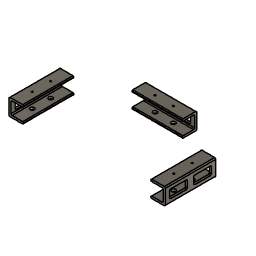
mac-holder v4 (Autodesk Fusion 360 design; units mm, degrees)
Autodesk Fusion 360 part; units mm, degrees
sketch "mac" plane through (0, 0, 0) normal (0, 0, 1) x (1, 0, 0)
  line L0 (0, 0) -> (355.6, 0)
  line L1 (355.6, 0) -> (355.6, 247.65)
  line L2 (355.6, 247.65) -> (0, 247.65)
  line L3 (0, 247.65) -> (0, 0)
  dimension "d1" = 355.6
  dimension "d2" = 247.65
  constraint horizontal L0
  constraint vertical L1
  constraint horizontal L2
  constraint vertical L3
  constraint coincident L0.start L3.end
  measures "d1" distance of L0.start L0.end
  measures "d2" distance of L0.start L2.end
extrude "Extrude1" add sketch "mac" along normal blind 19.05 makes body 1
sketch "front" plane through (0, 0, 0) normal (0, 1, 0) x (1, 0, 0)
  line L0 (0, 0) -> (0, -40)
  line L1 (0, -40) -> (35, -40)
  line L2 (35, -40) -> (35, -35)
  line L3 (35, -35) -> (5, -35)
  line L4 (5, -35) -> (5, -5)
  line L5 (5, -5) -> (35, -5)
  line L6 (35, -5) -> (35, 0)
  line L7 (35, 0) -> (0, 0)
  dimension "d5" = 5
  dimension "d6" = 5
  dimension "d7" = 5
  dimension "d8" = 30
  dimension "d9" = 35
  dimension "d10" = 35
  constraint coincident L0.start L7.end
  constraint vertical L0
  constraint perpendicular L0 L1
  constraint perpendicular L1 L2
  constraint perpendicular L0 L3
  constraint perpendicular L3 L4
  constraint perpendicular L4 L5
  constraint perpendicular L5 L6
  constraint perpendicular L0 L7
  measures "d5" distance of L5.end L6.end
  measures "d6" distance of L1.end L2.end
  measures "d7" distance of L0 L4
  measures "d8" distance of L3 L5
  measures "d9" distance of L6.end L0.start
  measures "d10" distance of L0.end L1.end
extrude "Extrude2" add sketch "front" along normal blind 120 separate body makes body 2
sketch "side" plane through (0, 0, 0) normal (-1, 0, 0) x (0, -1, 0)
  line L0 (0, 0) -> (0, 40)
  line L1 (0, 40) -> (-120, 40)
  line L2 (-120, 40) -> (-120, 0)
  line L3 (-120, 0) -> (0, 0)
  line L4 (-110, 10) -> (-10, 10)
  line L5 (-10, 10) -> (-10, 30)
  line L6 (-10, 30) -> (-110, 30)
  line L7 (-110, 30) -> (-110, 10)
  line L8 (-60, 30) -> (-60, 10) construction
  line L9 (-67.5, 30) -> (-67.5, 10)
  line L10 (-52.5, 30) -> (-52.5, 10)
  dimension "d13" = -10
  dimension "d14" = 7.5
  constraint midpoint L6 L8.start
  constraint midpoint L4 L8.end
  constraint coincident L6 L9.start
  constraint coincident L4 L9.end
  constraint perpendicular L4 L9
  constraint symmetric L8 L9.start L10.start
  constraint symmetric L8 L9.end L10.end
  measures "d14" distance of L8 L9
extrude "Extrude3" cut sketch "side" against normal up to surface (5 mm away) contours L4 L6 L7 L9 | L4 L5 L6 L10 bodies 2
fillet "Fillet1" radius 2.5 8 edges at (2.5, 52.5, 30) (2.5, 10, 30) (2.5, 10, 10) (2.5, 52.5, 10) (2.5, 67.5, 10) (2.5, 67.5, 30) (2.5, 110, 30) (2.5, 110, 10) on bodies 2
fillet "Fillet2" radius 2.5 2 edges at (0, 60, 40) (0, 60, 0) on bodies 2
fillet "Fillet3" radius 2.5 2 edges at (5, 60, 35) (5, 60, 5) on bodies 2
fillet "Fillet4" radius 2 4 edges at (35, 60, 40) (35, 60, 35) (35, 60, 5) (35, 60, 0) on bodies 2
sketch "top" plane through (0, 0, 40) normal (0, 0, 1) x (-1, 0, 0)
  line L0 (-33, 0) -> (-33, -120)
  line L1 (-33, -120) -> (-2.5, -120)
  line L2 (-2.5, -120) -> (-2.5, 0)
  line L3 (-2.5, 0) -> (-33, 0)
  line L4 (-33, -60) -> (-2.5, -60) construction
  line L5 (-17.75, -120) -> (-17.75, 0) construction
  circle A0 centre (-17.75, -38) radius 2
  circle A1 centre (-17.75, -82) radius 2
  circle A2 centre (-17.75, -38) radius 5
  circle A3 centre (-17.75, -82) radius 5
  circle A4 centre (-17.75, -38) radius 3
  circle A5 centre (-17.75, -82) radius 3
  dimension "d27" = 4
  dimension "d28" = 20
  dimension "d29" = 10
  dimension "d35" = 6
  constraint midpoint L0 L4.start
  constraint midpoint L2 L4.end
  constraint midpoint L1 L5.start
  constraint midpoint L3 L5.end
  constraint coincident L5 A0.centre
  constraint symmetric L4 A0 A1
  constraint concentric A0 A2
  constraint symmetric L4 A2 A3
  constraint concentric A0 A4
  constraint symmetric L4 A4 A5
  measures "d27" diameter of A0
  measures "d28" distance of L4 A0
  measures "d29" diameter of A2
  measures "d35" diameter of A4
extrude "Extrude4" cut sketch "top" against normal up to surface (40 mm away) contours A0 | A1 bodies 2
extrude "Extrude5" cut sketch "top" against normal up to surface (5 mm away) from surface at -35 contours A2 | A3 | A4 | A5 bodies 2
extrude "Extrude6" cut sketch "top" along normal blind 2 from surface at -5 contours A4 | A5 bodies 2
move_body "Move1" bodies 1 to x (1, 0, 0) y (0, 1, 0) z (0, 0, 1) at (9, 0, 10)
ref_plane "WorkPlane1" through (186.8, 123.825, 19.525) normal (1, 0, 0) x (0, 1, 0)
mirror "Mirror1" about plane through (186.8, 123.825, 19.525) normal (1, 0, 0) of bodies 2 makes body 3
fillet "Fillet5" radius 10 4 edges at (9, 0, 19.525) (364.6, 0, 19.525) (364.6, 247.65, 19.525) (9, 247.65, 19.525) on bodies 1
move_body "Move2" bodies 1 to x (1, 0, 0) y (0, 1, 0) z (0, 0, 1) at (0, -60, 0)
copy_body "CopyPasteBodies1" bodies 3 makes body 4
move_body "Move3" bodies 4 to x (0, 1, 0) y (-1, 0, 0) z (0, 0, 1) at (258.6, -178.6, 0)
move_body "Move4" bodies 4 to x (1, 0, 0) y (0, 1, 0) z (0, 0, 1) at (-5, 0, 0)
hidden bodies 1
named bodies: "mac", "mac-holder-left", "mac-holder-right", "mac-holder (1)", "mac-holder-back"
